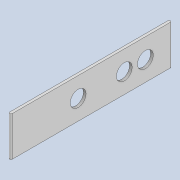
# Autodesk Inventor part: fin_12mm_h
Saved by Autodesk Inventor 2020 (Build 240168000, 168)
## iProperties
Created: 2021-10-03
Part Number: fin_12mm_h
Material: Generic
Document SubType Name: Modeling
Designer: Shuang Peng
Density: 1 g/cm^3
Appearance: Default
Author: Shuang Peng
Autodesk Inventor part; units mm, degrees
ref_plane "YZ Plane" through (0, 0, 0) normal (1, 0, 0) x (0, 1, 0)
ref_plane "XZ Plane" through (0, 0, 0) normal (0, 1, 0) x (-1, 0, 0)
ref_plane "XY Plane" through (0, 0, 0) normal (0, 0, 1) x (1, 0, 0)
sketch "Sketch1" plane through (0, 0, 0) normal (0, 1, 0) x (-1, 0, 0)
  line L0 (0, 0) -> (0, -12) construction
  line L1 (-0.1, 0) -> (-0.1, -12)
  line L2 (0.1, -12) -> (0.1, 0)
  arc A0 (0.1, 0) -> (-0.1, 0) centre (0, 0) ccw
  arc A1 (-0.1, -12) -> (0.1, -12) centre (0, -12) ccw
  point P0 (0, -6)
  dimension "d0" = 12
  dimension "d1" = 0.2
  constraints: 8 end point, 4 point on circle, 4 tangent, 2 centre point, 1 midpoint, 1 parallel, 1 vertical
  measures "d0" distance of L0.start L0.end
  measures "d1" diameter of A1
extrude "Extrusion1" add sketch "Sketch1" along normal blind 3
sketch "Sketch2" plane through (0.1, 0, 0) normal (1, 0, 0) x (0, 0, -1)
  line L0 (12.1, 0) -> (12.1, 3) projected
  line L1 (12.1, 1.5) -> (10.1, 1.5)
  circle A0 centre (10.1, 1.5) radius 0.6
  point P0 (0, 0)
  dimension "d4" = 2
  dimension "d5" = 1.2
  constraints: 2 end point, 1 centre point, 1 coincident, 1 horizontal, 1 midpoint
  measures "d4" distance of L1.start L1.end
  measures "d5" diameter of A0
extrude "Extrusion2" cut sketch "Sketch2" against normal blind 3
sketch "Sketch3" plane through (0.1, 0, 0) normal (1, 0, 0) x (0, 0, -1)
  line L0 (0, 0) -> (0, 3) projected
  line L1 (0, 1.5) -> (5, 1.5)
  line L2 (5, 1.5) -> (8.5, 1.5)
  circle A0 centre (5, 1.5) radius 0.6
  circle A1 centre (8.5, 1.5) radius 0.6
  dimension "d8" = 5
  dimension "d9" = 3.5
  dimension "d10" = 1.2
  dimension "d11" = 1.2
  constraints: 4 end point, 2 centre point, 2 coincident, 1 collinear, 1 horizontal, 1 midpoint
  measures "d8" distance of L1.start L1.end
  measures "d9" distance of L1.end L2.end
  measures "d10" diameter of A0
  measures "d11" diameter of A1
extrude "Extrusion3" cut sketch "Sketch3" against normal blind 10
body "Solid1"
